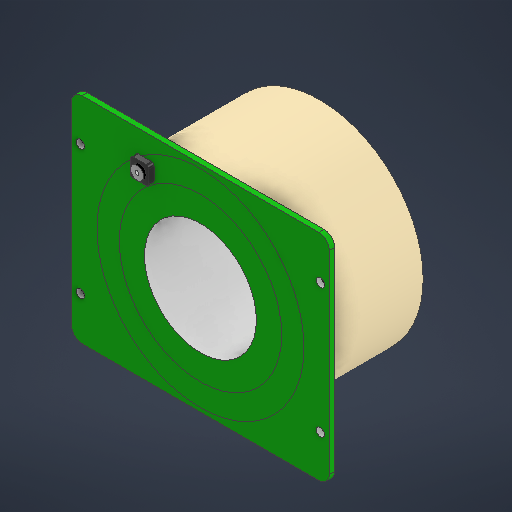
# Autodesk Inventor part: PCB
Saved by Autodesk Inventor 2026.1 (Build 301233000, 233)
## iProperties
Created: 2025-11-06
Part Number: PCB
Material: Generic
Document SubType Name: Modeling
Designer: SPEL
Density: 1 g/cm^3
Appearance: Default
Author: SPEL
Autodesk Inventor part; units mm, degrees
ref_plane "YZ Plane" through (0, 0, 0) normal (1, 0, 0) x (0, 1, 0)
ref_plane "XZ Plane" through (0, 0, 0) normal (0, 1, 0) x (-1, 0, 0)
ref_plane "XY Plane" through (0, 0, 0) normal (0, 0, 1) x (1, 0, 0)
sketch "Sketch1" plane through (0, 0, 0) normal (0, 0, 1) x (1, 0, 0)
  circle A0 centre (0, 0) radius 31
  line L0 (49.2, 41) -> (-49.2, 41)
  line L1 (-49.2, 41) -> (-49.2, -41)
  line L2 (-49.2, -41) -> (49.2, -41)
  line L3 (49.2, -41) -> (49.2, 41)
  line L4 (49.2, 41) -> (-49.2, -41) construction
  line L5 (-49.2, 41) -> (49.2, -41) construction
  line L6 (-37.7816, 31.4847) -> (-27.7816, 31.4847)
  line L7 (-27.7816, 31.4847) -> (-27.7816, 7.4847)
  line L8 (-27.7816, 7.4847) -> (-37.7816, 7.4847)
  line L9 (-37.7816, 7.4847) -> (-37.7816, 31.4847)
  line L10 (-37.7816, 7.4847) -> (-27.7816, 7.4847)
  line L11 (-27.7816, 7.4847) -> (-27.7816, 12.2304)
  line L12 (-27.7816, 12.2304) -> (-37.7816, 12.2304)
  line L13 (-37.7816, 12.2304) -> (-37.7816, 7.4847)
  circle A1 centre (-21.2061, 28.9956) radius 2.5
  line L14 (-17.7061, 32.4956) -> (-24.7061, 32.4956)
  line L15 (-24.7061, 32.4956) -> (-24.7061, 25.4956)
  line L16 (-24.7061, 25.4956) -> (-17.7061, 25.4956)
  line L17 (-17.7061, 25.4956) -> (-17.7061, 32.4956)
  line L18 (-17.7061, 32.4956) -> (-24.7061, 25.4956) construction
  line L19 (-24.7061, 32.4956) -> (-17.7061, 25.4956) construction
  circle A2 centre (-21.2061, 28.9956) radius 0.75
  line L20 (48.45, -20) -> (38.45, -20)
  line L21 (38.45, -20) -> (38.45, 20)
  line L22 (38.45, 20) -> (48.45, 20)
  line L23 (48.45, 20) -> (48.45, -20)
  circle A3 centre (-45.8, 24.7) radius 1.6
  circle A4 centre (-45.8, -24.7) radius 1.6
  circle A5 centre (45.8, -24.7) radius 1.6
  circle A6 centre (45.8, 24.7) radius 1.6
  point P0 (-37.7816, 12.2304)
  dimension "d0" = 62
  dimension "d1" = 98.4
  dimension "d2" = 82
  dimension "d6" = 10
  dimension "d7" = 24
  dimension "d16" = 5
  dimension "d17" = 7
  dimension "d18" = 7
  dimension "d21" = 1.5
  dimension "d29" = 82
  dimension "d33" = 40
  dimension "d34" = 10
  dimension "d35" = 21
  dimension "d39" = 0.75
  dimension "d40" = 7.45
  dimension "d50" = 3.2
  dimension "d52" = 3.2
  dimension "d53" = 3.2
  dimension "d55" = 3.2
  dimension "d57" = 49.4
  dimension "d58" = 49.4
  dimension "d59" = 91.6
  dimension "d60" = 91.6
  dimension "d61" = 45.8
  dimension "d62" = 45.8
  dimension "d63" = 24.7
  dimension "d64" = 24.7
  constraints: 48 end point, 10 parallel, 7 centre point, 5 horizontal, 5 perpendicular, 4 midpoint, 2 coincident, 2 point on line
  measures "d0" diameter of A0
  measures "d1" distance of L2.end L1.end
  measures "d2" distance of L1.end L0.end
  measures "d6" distance of L7.end L8.end
  measures "d7" distance of L6.end L7.end
  measures "d16" diameter of A1
  measures "d17" distance of L16.end L15.end
  measures "d18" distance of L15.end L14.end
  measures "d21" diameter of A2
  measures "d29" distance of L2.end L0.start
  measures "d33" distance of L22.end L20.start
  measures "d34" distance of L21.end L22.end
  measures "d35" distance between parallel lines of L2 L20
  measures "d39" distance between parallel lines of L23 L3
  measures "d40" distance edge to line of A0 L21
  measures "d50" diameter of A3
  measures "d52" diameter of A4
  measures "d53" diameter of A5
  measures "d55" diameter of A6
  measures "d57" distance of A4.centre A3.centre
  measures "d58" distance of A5.centre A6.centre
  measures "d59" distance of A6.centre A3.centre
  measures "d60" distance of A5.centre A4.centre
  measures "d61" horizontal distance of A3.centre point (0, 0)
  measures "d62" horizontal distance of point (0, 0) A4.centre
  measures "d63" vertical distance of point (0, 0) A3.centre
  measures "d64" vertical distance of point (0, 0) A6.centre
extrude "Extrusion1" add sketch "Sketch1" along normal blind 2 contours A0 L12 L9 L6 L7 | L8 L9 L12 A0 | L3 L2 L1 L0 | A1 | L17 L16 L15 L14 | A2 | L20 L21 L22 L23 | A3 | A4 | A5 | A6
fillet "Fillet1" radius 4 4 edges at (49.2, -41, 1) (49.2, 41, 1) (-49.2, -41, 1) (-49.2, 41, 1)
extrude "Extrusion5" add sketch "Sketch1" along normal blind 5 contours A1 | A2
extrude "Extrusion6" add sketch "Sketch1" along normal blind 4 contours L17 L16 L15 L14
extrude "Extrusion7" add sketch "Sketch1" along normal blind 5.1 contours A2
fillet "Fillet2" radius 0.1 1 edges at (-21.9561, 28.9956, 5.1)
fillet "Fillet3" radius 1 4 edges at (-24.7061, 32.4956, 3) (-24.7061, 25.4956, 3) (-17.7061, 32.4956, 3) (-17.7061, 25.4956, 3)
sketch "Sketch2" plane through (0, 0, 2) normal (0, 0, 1) x (1, 0, 0)
  circle A0 centre (0, 0) radius 39.5
  circle A1 centre (0, 0) radius 19.25
  circle A2 centre (0, 0) radius 21.35
  dimension "d41" = 79
  dimension "d44" = 38.5
  dimension "d45" = 42.7
  constraints: 3 centre point, 3 coincident
  measures "d41" diameter of A0
  measures "d44" diameter of A1
  measures "d45" diameter of A2
extrude "Extrusion10" add sketch "Sketch2" against normal blind 45.5 separate body contours A0
extrude "Extrusion11" cut sketch "Sketch2" against normal blind 40 contours A2 bodies 1
extrude "Extrusion12" cut sketch "Sketch2" against normal blind 40 contours A1 bodies 1
extrude "Extrusion13" cut sketch "Sketch1" along normal blind 100 contours A3 | A4 | A5 | A6 bodies 2 1
equation "\"d35\" = 0.5 * d29 - 0.5 * d33"
equation "\"d52\" = d50"
equation "\"d53\" = d54"
equation "\"d55\" = d56"
equation "\"d58\" = d57"
equation "\"d60\" = d59"
equation "\"d61\" = 0.5 * d59"
equation "\"d62\" = d61"
equation "\"d63\" = 0.5 * d57"
equation "\"d64\" = d63"
equation "\"d54\" = 3.2"
equation "\"d56\" = 3.2"
body "Solid1"
body "Solid3"
